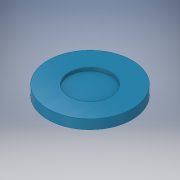
# Autodesk Inventor part: sensor1
Saved by Autodesk Inventor 2018 (Build 220112000, 112)
## iProperties
Created: 2021-03-17
Part Number: sensor1
Material: Generic
Document SubType Name: Modeling
Designer: Ramana Bharathi
Density: 0.60286 g/cm^3
Appearance: Sky Blue Dark
Mass: 25 g
Surface Area: 126.92 cm^2
Volume: 41.469 cm^3
Author: Ramana Bharathi
Autodesk Inventor part; units mm, degrees
ref_plane "YZ Plane" through (0, 0, 0) normal (1, 0, 0) x (0, 1, 0)
ref_plane "XZ Plane" through (0, 0, 0) normal (0, 1, 0) x (-1, 0, 0)
ref_plane "XY Plane" through (0, 0, 0) normal (0, 0, 1) x (1, 0, 0)
sketch "Sketch1" plane through (0, 0, 0) normal (0, 1, 0) x (-1, 0, 0)
  circle A0 centre (0, 0) radius 40
  dimension "d0" = 80
  constraints: 1 centre point, 1 coincident
  measures "d0" diameter of A0
extrude "Extrusion1" add sketch "Sketch1" along normal blind 9
sketch "Sketch3" plane through (0, 9, 0) normal (0, 1, 0) x (1, 0, 0)
  circle A0 centre (0, 0) radius 20
  dimension "d6" = 40
  constraints: 1 centre point, 1 coincident
  measures "d6" diameter of A0
extrude "Extrusion3" cut sketch "Sketch3" against normal blind 3
body "Solid1"
